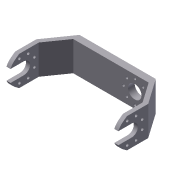
# Autodesk Inventor part: Hips
Saved by Autodesk Inventor 2011 (Build 150239000, 239)
## iProperties
Created: 2010-11-21
Part Number: Hips
Document SubType Name: Modeling
Designer: Milton
Density: 2.71 g/cm^3
Mass: 27.9597 g
Surface Area: 72.448 cm^2
Volume: 10.3172 cm^3
Material: Aluminum-6061
Author: Milton
Autodesk Inventor part; units mm, degrees
ref_plane "YZ Plane" through (0, 0, 0) normal (1, 0, 0) x (0, 1, 0)
ref_plane "XZ Plane" through (0, 0, 0) normal (0, 1, 0) x (-1, 0, 0)
ref_plane "XY Plane" through (0, 0, 0) normal (0, 0, 1) x (1, 0, 0)
sketch "Sketch1" plane through (0, 0, 0) normal (0, 0, 1) x (1, 0, 0)
  line L0 (26.7421, 25.9605) -> (26.7421, 49.1206)
  line L1 (40.2452, 62.9605) -> (96.239, 62.9605)
  line L2 (39.9339, 67.9605) -> (96.5503, 67.9605)
  line L3 (106.7421, 25.9605) -> (106.7421, 47.9605)
  line L4 (26.7421, 25.9605) -> (29.7421, 25.9605)
  line L5 (106.7421, 25.9605) -> (109.7421, 25.9605)
  line L6 (109.7421, 25.9605) -> (109.7421, 49.1206)
  line L7 (29.7421, 25.9605) -> (29.7421, 47.9605)
  line L8 (29.7421, 47.9605) -> (40.2452, 62.9605)
  line L9 (26.7421, 49.1206) -> (39.9339, 67.9605)
  line L10 (106.7421, 47.9605) -> (96.239, 62.9605)
  line L11 (109.7421, 49.1206) -> (96.5503, 67.9605)
  point P0 (0, 0)
  constraints: 24 end point
extrude "Extrusion1" add sketch "Sketch1" along normal blind 45
sketch "Sketch2" plane through (109.7421, 25.9605, 0) normal (1, 0, 0) x (0, 0, -1)
  line L0 (-45, 23.1601) -> (-45, 0) projected
  line L1 (0, 0) -> (-45, 0) projected
  line L2 (0, 23.1601) -> (0, 0) projected
  line L3 (0, 23.1601) -> (-45, 23.1601) projected
  line L4 (-45, 23.1601) -> (-31.3837, 4.513)
  line L5 (0, 23.1601) -> (-13.6163, 4.513)
  arc A0 (-18, 11) -> (-27, 11) centre (-22.5, 11) ccw
  line L6 (-45, 23.1601) -> (-45, -1.8399)
  line L7 (-45, -1.8399) -> (0, -1.8399)
  line L8 (0, -1.8399) -> (0, 23.1601)
  line L9 (-18, 11) -> (-18, 0.9626)
  line L10 (-27, 11) -> (-27, 0.9626)
  arc A1 (-18, 0.9626) -> (-13.6163, 4.513) centre (-22.5, 11) ccw
  arc A2 (-31.3837, 4.513) -> (-27, 0.9626) centre (-22.5, 11) ccw
  line L11 (-45, 42) -> (-33.5, 42)
  line L12 (-33.5, 42) -> (-33.5, 2)
  line L13 (-33.5, 2) -> (-45, 2)
  line L14 (-45, 2) -> (-45, 42)
  line L15 (0, 42) -> (-11.5, 42)
  line L16 (-11.5, 42) -> (-11.5, 2)
  line L17 (-11.5, 2) -> (0, 2)
  line L18 (0, 2) -> (0, 42)
  circle A3 centre (-22.5, 11) radius 11
  point P0 (0, -25.9605)
  dimension "d3" = 11
  dimension "d4" = 9
  dimension "d5" = 25
  dimension "d14" = 11.5
  dimension "d15" = 11.5
  dimension "d16" = 40
  dimension "d17" = 40
  constraints: 30 end point, 6 parallel, 6 point on circle, 4 perpendicular, 4 tangent, 3 centre point, 2 coincident, 2 horizontal, 3 other
  measures "d3" distance from line of A1.centre L1
  measures "d4" diameter of A0
  measures "d5" distance of L0.start L6.end
  measures "d14" distance of L12.end L13.end
  measures "d15" distance between parallel lines of L18 L16
  measures "d16" distance of L11.end L12.end
  measures "d17" distance of L15.end L16.end
sketch "Sketch3" plane through (39.9339, 67.9605, 0) normal (0, 1, 0) x (1, 0, 0)
  circle A0 centre (46.0082, -22.5) radius 5
  line L0 (69.8082, 0) -> (69.8082, -45) projected
  point P0 (-39.9339, 0)
  dimension "d8" = 10
  dimension "d9" = 23.8
  constraints: 1 centre point
  measures "d8" diameter of A0
  measures "d9" distance from line of L0 A0.centre
extrude "Extrusion3" cut sketch "Sketch3" against normal blind 45
extrude "Extrusion4" cut sketch "Sketch2" against normal through all contours L4 L12 L13 L0 | L14 L11 L12 L3 | L3 L12 L4 | L13 L12 L4 A2 A3 L1 L0 | L16 L15 L18 L3 | L3 L5 L16 | A3 A1 L5 L16 L17 L2 L1 | A3 L10 A0 L9 | L2 L17 L16 L5
sketch "Sketch4" plane through (109.7421, 33.3718, 33.5) normal (1, 0, 0) x (0, 0, -1)
  arc A0 (15.5, -6.4487) -> (19.8837, -2.8983) centre (11, 3.5887) ccw projected
  line L0 (11, 3.5887) -> (19.5, 3.5887) construction
  circle A1 centre (7.7472, 11.4417) radius 1
  point P0 (33.5, -33.3718)
  dimension "d22" = 2
  constraints: 2 end point, 1 centre point, 1 horizontal
  measures "d22" diameter of A1
extrude "Extrusion5" cut sketch "Sketch4" against normal through all
pattern_circular "Circular Pattern1" count 8 over 360 about axis through (109.7421, 36.9605, 22.5) along (-1, 0, 0) of "Extrusion5"
sketch "Sketch5" plane through (40.2452, 62.9605, 11.5) normal (0, -1, 0) x (1, 0, 0)
  circle A0 centre (45.6969, 11) radius 5 projected
  circle A1 centre (37.1969, 11) radius 1
  point P0 (-40.2452, -11.5)
  dimension "d28" = 2
  dimension "d29" = 8.5
  constraints: 1 centre point
  measures "d28" diameter of A1
  measures "d29" distance of A0.centre A1.centre
extrude "Extrusion6" cut sketch "Sketch5" against normal through all contours A1
pattern_circular "Circular Pattern2" count 8 over 360 about axis through (85.9421, 67.9605, 22.5) along (0, -1, 0) of "Extrusion6"
body "Solid1"
